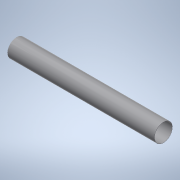
# Autodesk Inventor part: Tubo tolba
Saved by Autodesk Inventor 2020 (Build 240168000, 168)
## iProperties
Created: 2020-02-16
Part Number: Tubo tolba
Material: Steel, Mild, Welded
Document SubType Name: Modeling
Designer: PabloGod
Density: 7.85 g/cm^3
Appearance: Weld - Steel Mild
Author: PabloGod
Autodesk Inventor part; units mm, degrees
ref_plane "YZ Plane" through (0, 0, 0) normal (1, 0, 0) x (0, 1, 0)
ref_plane "XZ Plane" through (0, 0, 0) normal (0, 1, 0) x (-1, 0, 0)
ref_plane "XY Plane" through (0, 0, 0) normal (0, 0, 1) x (1, 0, 0)
sketch "Boceto1" plane through (0, 0, 0) normal (1, 0, 0) x (0, 1, 0)
  circle A0 centre (0, 0) radius 60
  circle A1 centre (0, 0) radius 62
  line L0 (0, 0) -> (1013.9731, 0) construction
  dimension "d0" = 120
  dimension "d1" = 124
  constraints: 2 centre point, 2 coincident, 2 end point, 1 horizontal
  measures "d0" diameter of A0
  measures "d1" diameter of A1
extrude "Extrusión1" add sketch "Boceto1" along normal blind 1000
